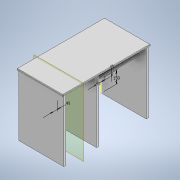
# Autodesk Inventor part: Work Table
Saved by Autodesk Inventor 2020 (Build 240168000, 168)
## iProperties
Created: 2021-01-02
Part Number: Work Table
Material: Generic
Document SubType Name: Modeling
Designer: frost
Density: 1 g/cm^3
Appearance: Default
Author: frost
Autodesk Inventor part; units mm, degrees
ref_plane "YZ Plane" through (0, 0, 0) normal (1, 0, 0) x (0, 1, 0)
ref_plane "XZ Plane" through (0, 0, 0) normal (0, 1, 0) x (-1, 0, 0)
ref_plane "XY Plane" through (0, 0, 0) normal (0, 0, 1) x (1, 0, 0)
sketch "Sketch1" plane through (0, 0, 0) normal (0, 1, 0) x (-1, 0, 0)
  line L0 (280, 535) -> (-280, 535)
  line L1 (-280, 535) -> (-280, -535)
  line L2 (-280, -535) -> (280, -535)
  line L3 (280, -535) -> (280, 535)
  line L4 (280, 535) -> (-280, -535) construction
  line L5 (-280, 535) -> (280, -535) construction
  point P0 (0, 0)
  dimension "d0" = 560
  dimension "d1" = 1070
  constraints: 12 end point, 2 midpoint, 2 parallel, 1 horizontal, 1 perpendicular
  measures "d0" distance of L2.end L1.end
  measures "d1" distance of L1.end L0.end
extrude "Extrusion1" add sketch "Sketch1" along normal blind 20
fillet "Fillet1" radius 5 12 edges at (280, 20, 0) (0, 20, -535) (280, 0, 0) (0, 20, 535) (-280, 20, 0) (-280, 0, 0) (0, 0, 535) (0, 0, -535) (280, 10, -535) (280, 10, 535) (-280, 10, -535) (-280, 10, 535)
sketch "Sketch2" plane through (0, 0, 0) normal (0, -1, 0) x (1, 0, 0)
  line L0 (275, 515) -> (-275, 515)
  line L1 (-275, 515) -> (-275, 490)
  line L2 (-275, 490) -> (275, 490)
  line L3 (275, 490) -> (275, 515)
  line L4 (-280, 530) -> (-280, -530) projected
  line L5 (280, -530) -> (280, 530) projected
  line L6 (275, 535) -> (-275, 535) projected
  point P0 (0, 0)
  dimension "d5" = 5
  dimension "d6" = 5
  dimension "d7" = 20
  dimension "d8" = 25
  constraints: 8 end point, 2 parallel, 1 horizontal, 1 perpendicular
  measures "d5" distance between parallel lines of L4 L1
  measures "d6" distance between parallel lines of L5 L3
  measures "d7" distance between parallel lines of L6 L0
  measures "d8" distance of L2.end L0.start
extrude "Extrusion2" add sketch "Sketch2" along normal blind 750
ref_plane "Work Plane1" through (-275, 5, 0) normal (0, 0, 1) x (1, 0, 0)
mirror "Mirror1" about plane through (-275, 5, 0) normal (0, 0, 1) of "Extrusion2"
ref_plane "Work Plane2" through (275, 0, 303) normal (0, 0, -1) x (-1, 0, 0)
mirror "Mirror2" about plane through (275, 0, 303) normal (0, 0, -1) of "Extrusion2"
sketch "Sketch3" plane through (-275, -750, 91) normal (-1, 0, 0) x (0, 0, 1)
  line L0 (-606, 750) -> (-621, 750) projected
  line L1 (25, 750) -> (25, 0) projected
  line L2 (-606, 750) -> (25, 750)
  line L3 (25, 750) -> (25, 150)
  line L4 (25, 150) -> (-606, 150)
  line L5 (-606, 150) -> (-606, 750)
  line L6 (-606, 0) -> (-581, 0) projected
  line L7 (-536, 750) -> (-45, 750)
  line L8 (-45, 750) -> (-45, 195)
  line L9 (-45, 195) -> (-536, 195)
  line L10 (-536, 195) -> (-536, 750)
  line L11 (-581, 750) -> (-581, 0) projected
  line L12 (0, 750) -> (0, 0) projected
  point P0 (-91, 750)
  point P1 (-581, 150)
  point P2 (0, 150)
  dimension "d12" = 150
  dimension "d13" = 45
  dimension "d14" = 45
  dimension "d15" = 45
  constraints: 16 end point, 4 parallel, 2 horizontal, 2 perpendicular, 2 point on line
  measures "d12" distance between parallel lines of L6 L4
  measures "d13" distance between parallel lines of L4 L9
  measures "d14" distance between parallel lines of L11 L10
  measures "d15" distance between parallel lines of L12 L8
extrude "Extrusion3" add sketch "Sketch3" along normal blind 20
extrude "Extrusion4" add sketch "Sketch3" against normal blind 35 contours L12 L4 L11 L2 L10 L9 L8
sketch "Sketch4" plane through (-240, -750, 91) normal (1, 0, 0) x (0, 0, -1)
  line L0 (25, 660) -> (559.852, 660)
  line L1 (584.852, 660) -> (584.852, 645)
  line L2 (559.852, 645) -> (25, 645)
  line L3 (25, 645) -> (25, 660)
  line L4 (0, 750) -> (581, 750) projected
  line L5 (559.852, 660) -> (559.852, 645)
  line L6 (0, 750) -> (0, 0) projected
  point P0 (91, 750)
  dimension "d20" = 90
  dimension "d21" = 15
  dimension "d22" = 25
  dimension "d23" = 25
  constraints: 10 end point, 2 parallel, 1 horizontal, 1 perpendicular, 1 vertical
  measures "d20" distance between parallel lines of L4 L0
  measures "d21" distance of L2.end L0.start
  measures "d22" distance between parallel lines of L1 L5
  measures "d23" distance between parallel lines of L6 L3
extrude "Extrusion5" add sketch "Sketch4" along normal blind 450
body "Solid1"
